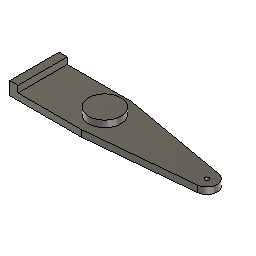
marking-jig-1.5mm (Autodesk Fusion 360 design; units mm, degrees)
Autodesk Fusion 360 part; units mm, degrees
sketch "jig" plane through (0, 0, 0) normal (0, 0, 1) x (1, 0, 0)
  line L0 (0, 0) -> (21.68, 0)
  line L1 (22.0268, 15) -> (0, 15)
  line L2 (0, 15) -> (0, 0)
  line L3 (0, 0) -> (2.5, 0)
  line L4 (2.5, 0) -> (2.5, 15)
  line L5 (2.5, 15) -> (0, 15)
  line L6 (0, 15) -> (0, 0)
  line L7 (2.5, 7.5) -> (21.4, 7.5) construction
  circle A0 centre (21.4, 7.5) radius 4.995
  line L8 (21.4, 7.5) -> (53.8, 7.5) construction
  line L9 (53.8, 7.5) -> (53.8, 6.161) construction
  circle A1 centre (53.8, 6.161) radius 0.625
  line L10 (21.8035, 2.5213) -> (53.8586, 5.5388) construction
  line L11 (22.2769, 12.4174) -> (53.9097, 6.7763) construction
  line L12 (22.0268, 15) -> (54.2632, 9.2512)
  line L13 (21.68, 0) -> (54.0101, 3.0433)
  arc A2 (54.0101, 3.0433) -> (54.2632, 9.2512) centre (53.8, 6.161) ccw
  dimension "d2" = 15
  dimension "d3" = 2.5
  dimension "d4" = 18.9
  dimension "d5" = 9.99
  dimension "d6" = 32.4
  dimension "d7" = 1.339
  dimension "d8" = 1.25
  constraint horizontal L0
  constraint horizontal L1
  constraint vertical L2
  constraint coincident L0.start L2.end
  constraint horizontal L3
  constraint vertical L4
  constraint horizontal L5
  constraint vertical L6
  constraint midpoint L4 L7.start
  constraint perpendicular L4 L7
  constraint coincident L7.end A0.centre
  constraint parallel L7 L8
  constraint perpendicular L8 L9
  constraint coincident L9.end A1.centre
  constraint coincident A0 L10.start
  constraint coincident A1 L10.end
  constraint tangent A1 L10
  constraint coincident A0 L11.start
  constraint coincident A1 L11.end
  constraint tangent A1 L11
  constraint tangent A0 L11
  constraint parallel L11 L12
  constraint parallel L10 L13
  measures "d2" distance of L0.start L1.end
  measures "d3" distance of L0.start L3.end
  measures "d4" distance of L7.start L7.end
  measures "d5" diameter of A0
  measures "d6" distance of L7.end L8.end
  measures "d7" distance of L8.end L9.end
  measures "d8" diameter of A1
extrude "Extrude1" add sketch "jig" along normal blind 2 contours L0 L1 L2 L3 L4 L5 L6 | A0 makes body 1 at (0.8333, 10, 0) makes body 2 at (23.857, 6.5592, 0)
extrude "Extrude2" add sketch "jig" against normal blind 2 contours L0 L1 L2 L3 L4 L5 L6 | L0 L1 L4 L12 L13 A2 | A0 bodies 1 2
sketch "text" plane through (0, 0, -2) normal (0, 0, -1) x (1, 0, 0)
  circle A0 centre (53.8, -6.161) radius 0.625
  line L0 (0, -15) -> (22.0268, -15)
  line L1 (22.0268, -15) -> (54.2632, -9.2512)
  arc A1 (54.2632, -9.2512) -> (54.0101, -3.0433) centre (53.8, -6.161) ccw
  line L2 (54.0101, -3.0433) -> (21.68, 0)
  line L3 (21.68, 0) -> (0, 0)
  line L4 (0, 0) -> (0, -15)
  line L5 (22, -5) -> (10.0088, -5) construction
  line L6 (10.0088, -5) -> (10.0088, -11) construction
  line L7 (10.0088, -11) -> (22, -11) construction
  line L8 (22, -11) -> (22, -5) construction
  line L9 (6.5378, -10.9721) -> (5.4173, -9.0313)
  line L10 (7.6583, -9.0313) -> (6.5378, -10.9721)
  line L11 (6.25, -9.0313) -> (6.25, -4.3533)
  line L12 (6.25, -4.3533) -> (6.75, -4.3533)
  line L13 (6.75, -4.3533) -> (6.75, -9.0313)
  line L14 (5.4173, -9.0313) -> (6.25, -9.0313)
  line L15 (6.75, -9.0313) -> (7.6583, -9.0313)
  point P0 (6.5, -7)
  dimension "d17" = 0.5
  text T0 "TOP " font "Arial" height 6 bold align ink ink in box 0 x 0 at (22, -5) x (-1, 0) y (0, -1) spacing 1 kerned height is em
  constraint perpendicular L5 L6
  constraint parallel L5 L7
  constraint parallel L6 L8
  constraint equal L9 L10
  constraint parallel L11 L13
  constraint collinear L14 L15
  measures "d17" distance of L11.end L12.end
extrude "Extrude3" cut sketch "text" against normal blind 0.5 text T0 bodies 1
extrude "Extrude4" cut sketch "text" against normal blind 0.5 contours L9 L10 L11 L12 L13 L14 L15 bodies 1
move_face "OffsetFaces1" offset -0.1 1 faces at (26.3888, 7.251, 1.3333) on bodies 1
named bodies: "jig"
